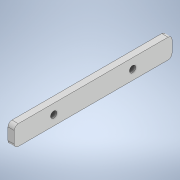
# Autodesk Inventor part: mocowanie zawieszenia
Saved by Autodesk Inventor 2021 (Build 250183000, 183)
## iProperties
Created: 2021-06-22
Part Number: mocowanie zawieszenia
Material: Generic
Document SubType Name: Modeling
Designer: Łukasz
Density: 1 g/cm^3
Appearance: Default
Author: Łukasz
Autodesk Inventor part; units mm, degrees
ref_plane "YZ Plane" through (0, 0, 0) normal (1, 0, 0) x (0, 1, 0)
ref_plane "XZ Plane" through (0, 0, 0) normal (0, 1, 0) x (-1, 0, 0)
ref_plane "XY Plane" through (0, 0, 0) normal (0, 0, 1) x (1, 0, 0)
sketch "Sketch1" plane through (0, 0, 0) normal (0, 0, 1) x (1, 0, 0)
  line L0 (0, 0) -> (8, 0)
  line L1 (8, 0) -> (8, 25)
  line L2 (8, 25) -> (0, 25)
  line L3 (0, 25) -> (0, 0)
  dimension "d0" = 8
  dimension "d1" = 25
  constraints: 8 end point, 2 parallel, 1 horizontal, 1 perpendicular
  measures "d0" distance of L2.end L1.end
  measures "d1" distance of L1.end L0.end
extrude "Extrusion1" add sketch "Sketch1" along normal blind 200
fillet "Fillet1" radius 5 4 edges at (4, 25, 200) (4, 0, 200) (4, 25, 0) (4, 0, 0)
sketch "Sketch2" plane through (8, 5, 0) normal (1, 0, 0) x (0, 0, -1)
  circle A0 centre (-50, 7.5) radius 4
  circle A1 centre (-150, 7.5) radius 4
  line L0 (-200, 0) -> (-200, 15) projected
  line L1 (0, 0) -> (0, 15) projected
  point P0 (0, -5)
  dimension "d5" = 8
  dimension "d6" = 8
  dimension "d9" = 50
  dimension "d10" = 50
  constraints: 2 centre point
  measures "d5" diameter of A0
  measures "d6" diameter of A1
  measures "d9" distance from line of L0 A1.centre
  measures "d10" distance from line of L1 A0.centre
extrude "Extrusion2" cut sketch "Sketch2" against normal up to surface (8 mm away)
body "Solid1"
